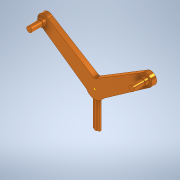
# Autodesk Inventor part: Gripper Base
Saved by Autodesk Inventor 2020 (Build 240168000, 168)
## iProperties
Created: 2021-06-06
Part Number: Gripper Base
Material: Gold
Document SubType Name: Modeling
Designer: ugwue
Density: 19.3 g/cm^3
Appearance: Metal 1600F Hot
Author: ugwue
Autodesk Inventor part; units mm, degrees
ref_plane "YZ Plane" through (0, 0, 0) normal (1, 0, 0) x (0, 1, 0)
ref_plane "XZ Plane" through (0, 0, 0) normal (0, 1, 0) x (-1, 0, 0)
ref_plane "XY Plane" through (0, 0, 0) normal (0, 0, 1) x (1, 0, 0)
sketch "Sketch1" plane through (0, 0, 0) normal (0, 0, 1) x (1, 0, 0)
  arc A0 (44.3036, 23.0175) -> (39.2001, 31.3912) centre (42.588, 27.714) ccw
  arc A1 (-39.2001, 31.3912) -> (-44.3036, 23.0175) centre (-42.588, 27.714) ccw
  arc A2 (-6.666, -3.4373) -> (6.666, -3.4373) centre (0, 0) ccw
  line L0 (0, 7.5) -> (39.2001, 31.3912)
  line L1 (6.666, -3.4373) -> (44.3036, 23.0175)
  line L2 (0, 7.5) -> (-39.2001, 31.3912)
  line L3 (-6.666, -3.4373) -> (-44.3036, 23.0175)
  dimension "d5" = 10
  dimension "d6" = 10
  dimension "d7" = 15
  constraints: 8 end point, 6 point on circle, 3 centre point, 1 coincident
  measures "d5" diameter of A0
  measures "d6" diameter of A1
  measures "d7" diameter of A2
extrude "Extrusion1" add sketch "Sketch1" along normal blind 4
fillet "Fillet1" radius 2 1 edges at (0, 7.5, 2)
sketch "Sketch2" plane through (0, 0, 4) normal (0, 0, 1) x (1, 0, 0)
  arc A0 (44.3036, 23.0175) -> (39.2001, 31.3912) centre (42.588, 27.714) ccw projected
  circle A1 centre (42.588, 27.714) radius 2.25
  arc A2 (-39.2001, 31.3912) -> (-44.3036, 23.0175) centre (-42.588, 27.714) ccw projected
  circle A3 centre (-42.588, 27.714) radius 2.25
  point P0 (0, 0)
  dimension "d11" = 4.5
  dimension "d12" = 4.5
  constraints: 2 centre point, 2 coincident
  measures "d11" diameter of A1
  measures "d12" diameter of A3
extrude "Extrusion2" add sketch "Sketch2" along normal blind 12
sketch "Sketch3" plane through (0, 0, 4) normal (0, 0, 1) x (1, 0, 0)
  arc A0 (44.3036, 23.0175) -> (39.2001, 31.3912) centre (42.588, 27.714) ccw projected
  circle A1 centre (42.588, 27.714) radius 2.75
  circle A2 centre (-42.588, 27.714) radius 2.25 projected
  circle A3 centre (-42.588, 27.714) radius 2.75
  point P0 (0, 0)
  dimension "d15" = 5.5
  dimension "d16" = 5.5
  constraints: 2 centre point, 2 coincident
  measures "d15" diameter of A1
  measures "d16" diameter of A3
extrude "Extrusion3" add sketch "Sketch3" along normal blind 3 contours A1 | A2 | A3
sketch "Sketch4" plane through (0, 0, 0) normal (0, 1, 0) x (-1, 0, 0)
  line L0 (2.5, 1.25) -> (-2.5, 1.25)
  line L1 (-2.5, 1.25) -> (-2.5, 2.75)
  line L2 (-2.5, 2.75) -> (2.5, 2.75)
  line L3 (2.5, 2.75) -> (2.5, 1.25)
  line L4 (2.5, 1.25) -> (-2.5, 2.75) construction
  line L5 (-2.5, 1.25) -> (2.5, 2.75) construction
  line L6 (-0.75, 0.5) -> (-0.75, 3.5)
  line L7 (-0.75, 3.5) -> (0.75, 3.5)
  line L8 (0.75, 3.5) -> (0.75, 0.5)
  line L9 (0.75, 0.5) -> (-0.75, 0.5)
  line L10 (-0.75, 0.5) -> (0.75, 3.5) construction
  line L11 (-0.75, 3.5) -> (0.75, 0.5) construction
  point P0 (0, 0)
  point P1 (0, 2)
  point P2 (0, 2)
  point P3 (-0.75, 2.75)
  point P4 (-0.75, 1.25)
  point P5 (0.75, 1.25)
  point P6 (0.75, 2.75)
  dimension "d19" = 5
  dimension "d20" = 1.5
  dimension "d21" = 3
  dimension "d22" = 1.5
  constraints: 24 end point, 5 midpoint, 5 parallel, 2 perpendicular, 1 horizontal
  measures "d19" distance of L0.start L0.end
  measures "d20" distance of L0.end L1.end
  measures "d21" distance of L6.start L6.end
  measures "d22" distance of L6.end L7.end
extrude "Extrusion4" add sketch "Sketch4" against normal blind 30
sketch "Sketch5" plane through (0, 0, 4) normal (0, 0, 1) x (1, 0, 0)
  point P0 (0, 0)
sketch "Sketch6" plane through (0, -30, 0) normal (0, -1, 0) x (1, 0, 0)
  point P0 (0, 0)
body "Solid1"
